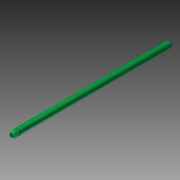
# Autodesk Inventor part: piston core
Saved by Autodesk Inventor 2012 (Build 160160000, 160)
## iProperties
Created: 2011-12-02
Part Number: piston core
Material: Default
Document SubType Name: Modeling
Designer: Antonella
Density: 1 g/cm^3
Author: Antonella
Autodesk Inventor part; units mm, degrees
ref_plane "YZ Plane" through (0, 0, 0) normal (1, 0, 0) x (0, 1, 0)
ref_plane "XZ Plane" through (0, 0, 0) normal (0, 1, 0) x (-1, 0, 0)
ref_plane "XY Plane" through (0, 0, 0) normal (0, 0, 1) x (1, 0, 0)
sketch "Sketch1" plane through (0, 0, 0) normal (0, 0, 1) x (1, 0, 0)
  circle A0 centre (0, 0) radius 3.175
  dimension "d0" = 6.35
  constraints: 1 centre point, 1 coincident
  measures "d0" diameter of A0
extrude "Extrusion1" add sketch "Sketch1" along normal mid plane 152.4
sketch "Sketch2" plane through (0, 0, 76.2) normal (0, 0, 1) x (1, 0, 0)
  circle A0 centre (0, 0) radius 3.175 projected
  line L0 (-1.508, 2.794) -> (-1.508, -2.794)
  line L1 (1.508, 2.794) -> (1.508, -2.794)
  line L2 (1.508, -2.794) -> (-1.508, -2.794)
  line L3 (-1.508, 2.794) -> (1.508, 2.794)
  dimension "d3" = 5.588
  constraints: 8 end point, 4 point on circle, 2 parallel, 1 perpendicular, 1 vertical
  measures "d3" distance of L1.start L1.end
extrude "Extrusion2" add sketch "Sketch2" along normal blind 6.35 contours L1 L2 L0 L3
sketch "Sketch3" plane through (1.508, -2.794, 76.2) normal (1, 0, 0) x (0, 0, -1)
  line L0 (-6.35, 5.588) -> (-6.35, 0) projected
  line L1 (0, 0) -> (-6.35, 0) projected
  line L2 (0, 5.588) -> (0, 0) projected
  line L3 (0, 5.588) -> (-6.35, 5.588) projected
  arc A0 (-3.556, 5.588) -> (-3.556, 0) centre (-3.556, 2.794) ccw
  point P0 (76.2, 2.794)
  constraints: 3 tangent, 2 point on circle, 2 point on line, 1 centre point
extrude "Extrusion3" cut sketch "Sketch3" against normal blind 6.35 contours L3 A0 L0 | A0 L1 L0
body "Solid1"
